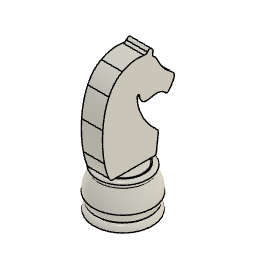
Knight (Autodesk Fusion 360 design; units mm, degrees)
Autodesk Fusion 360 part; units mm, degrees
sketch "Knight" plane through (0, 0, 0) normal (1, 0, 0) x (0, 1, 0)
  spline S0 degree 3 poles (14.2382, 40.3861) (12.0362, 41.9597) (10.374, 43.9521) (9.2277, 46.3988) knots 0 0 0 0 1 1 1 1
  spline S1 degree 3 poles (9.2277, 46.3988) (8.9049, 47.0874) (8.5729, 47.8295) (7.965, 48.2978) knots 0 0 0 0 1 1 1 1
  spline S2 degree 3 poles (7.965, 48.2978) (7.322, 48.7926) (6.9635, 49.21) (7.2909, 50.0977) knots 0 0 0 0 1 1 1 1
  spline S3 degree 3 poles (7.2909, 50.0977) (7.5575, 50.8193) (7.0766, 51.5377) (6.5098, 51.8929) knots 0 0 0 0 1 1 1 1
  spline S4 degree 3 poles (6.5098, 51.8929) (6.0189, 52.2004) (5.6055, 51.6131) (5.2649, 51.2248) knots 0 0 0 0 1 1 1 1
  spline S5 degree 3 poles (5.2649, 51.2248) (4.9137, 50.8259) (4.5287, 50.7565) (3.9698, 50.8517) knots 0 0 0 0 1 1 1 1
  spline S6 degree 3 poles (3.9698, 50.8517) (1.1063, 51.3405) (-1.6216, 50.8722) (-4.19, 49.5063) knots 0 0 0 0 1 1 1 1
  spline S7 degree 3 poles (-4.19, 49.5063) (-6.5984, 48.2257) (-8.1905, 46.2387) (-9.3084, 43.7854) knots 0 0 0 0 1 1 1 1
  spline S8 degree 3 poles (-9.3084, 43.7854) (-10.7411, 40.6434) (-11.4078, 37.3236) (-11.6307, 33.9177) knots 0 0 0 0 1 1 1 1
  spline S9 degree 3 poles (-11.6307, 33.9177) (-11.8748, 30.1792) (-11.7194, 26.4399) (-10.9898, 22.7563) knots 0 0 0 0 1 1 1 1
  spline S10 degree 3 poles (-10.9898, 22.7563) (-10.5982, 20.7798) (-10.1094, 18.8252) (-9.2118, 16.9824) knots 0 0 0 0 1 1 1 1
  spline S11 degree 3 poles (-9.2118, 16.9824) (-8.9036, 16.3467) (-8.5345, 16.0279) (-7.9848, 15.9194) knots 0 0 0 0 1 1 1 1
  line L0 (-7.9848, 15.9194) -> (7.9848, 15.9194)
  spline S12 degree 3 poles (7.9848, 15.9194) (8.4134, 16.0087) (8.5894, 16.2912) (8.6456, 16.8151) knots 0 0 0 0 1 1 1 1
  spline S13 degree 3 poles (8.6456, 16.8151) (8.8645, 18.8087) (9.1013, 20.7997) (9.3599, 22.7874) knots 0 0 0 0 1 1 1 1
  spline S14 degree 3 poles (9.3599, 22.7874) (9.4354, 23.3642) (9.264, 23.7505) (8.8347, 24.1526) knots 0 0 0 0 1 1 1 1
  spline S15 degree 3 poles (8.8347, 24.1526) (6.8755, 25.9809) (5.0611, 27.9362) (3.7779, 30.3254) knots 0 0 0 0 1 1 1 1
  spline S16 degree 3 poles (3.7779, 30.3254) (2.4874, 32.7311) (1.4793, 35.2208) (1.3887, 37.9983) knots 0 0 0 0 1 1 1 1
  spline S17 degree 3 poles (1.3887, 37.9983) (1.3742, 38.4243) (1.4688, 38.9918) (1.8332, 39.0242) knots 0 0 0 0 1 1 1 1
  spline S18 degree 3 poles (1.8332, 39.0242) (2.3214, 39.0678) (2.2076, 38.4659) (2.2751, 38.1147) knots 0 0 0 0 1 1 1 1
  spline S19 degree 3 poles (2.2751, 38.1147) (2.7103, 35.832) (3.9916, 35.1031) (6.2868, 35.656) knots 0 0 0 0 1 1 1 1
  spline S20 degree 3 poles (6.2868, 35.656) (8.2791, 36.1356) (10.2853, 36.4577) (11.9641, 34.6791) knots 0 0 0 0 1 1 1 1
  spline S21 degree 3 poles (11.9641, 34.6791) (12.1851, 34.4449) (12.914, 33.802) (13.5, 34.7611) knots 0 0 0 0 1 1 1 1
  spline S22 degree 3 poles (13.5, 34.7611) (13.9842, 35.5509) (14.6093, 36.2633) (15.0068, 37.1232) knots 0 0 0 0 1 1 1 1
  spline S23 degree 3 poles (15.0068, 37.1232) (15.6855, 38.5903) (15.5314, 39.4614) (14.2382, 40.3861) knots 0 0 0 0 1 1 1 1
  line L1 (-9.0666, 13.7263) -> (9.0666, 13.7263)
  spline S24 degree 3 poles (9.0666, 13.7263) (9.5051, 14.0021) (9.8597, 14.3719) (9.6268, 15.0432) knots 0 0 0 0 1 1 1 1
  spline S25 degree 3 poles (9.6268, 15.0432) (9.3398, 15.8694) (8.6274, 15.9131) (7.9084, 15.9117) knots 0 0 0 0 1 1 1 1
  spline S26 degree 3 poles (7.9084, 15.9117) (7.7682, 15.9117) (7.6299, 15.9064) (7.4897, 15.9078) knots 0 0 0 0 1 1 1 1
  spline S27 degree 3 poles (7.4897, 15.9078) (4.0157, 15.9117) (0.5404, 15.9223) (-2.9342, 15.9203) knots 0 0 0 0 1 1 1 1
  spline S28 degree 3 poles (-2.9342, 15.9203) (-4.7446, 15.9197) (-6.5551, 15.8932) (-8.3655, 15.8886) knots 0 0 0 0 1 1 1 1
  spline S29 degree 3 poles (-8.3655, 15.8886) (-9.1837, 15.8879) (-9.779, 15.5235) (-9.7836, 14.696) knots 0 0 0 0 1 1 1 1
  spline S30 degree 3 poles (-9.7836, 14.696) (-9.7863, 14.1403) (-9.4853, 13.8572) (-9.0666, 13.7263) knots 0 0 0 0 1 1 1 1
  line L2 (5.9758, 2.6224) -> (0, 2.6224)
  spline S31 degree 3 poles (10.1774, 0.0003) (10.5042, 0.001) (10.8839, -0.1015) (11.0042, 0.4012) knots 0 0 0 0 1 1 1 1
  spline S32 degree 3 poles (11.0042, 0.4012) (11.2509, 1.4258) (10.3401, 2.6177) (9.2877, 2.6158) knots 0 0 0 0 1 1 1 1
  line L3 (8.8867, 13.7263) -> (-8.8867, 13.7263)
  spline S33 degree 3 poles (-8.8867, 13.7263) (-9.3246, 13.5212) (-9.6474, 13.0919) (-9.9642, 12.5826) knots 0 0 0 0 1 1 1 1
  spline S34 degree 3 poles (-9.9642, 12.5826) (-10.3082, 12.0296) (-10.5734, 11.4515) (-10.8644, 10.8807) knots 0 0 0 0 1 1 1 1
  spline S35 degree 3 poles (-10.8644, 10.8807) (-12.108, 8.4578) (-11.977, 6.0381) (-10.8883, 3.5947) knots 0 0 0 0 1 1 1 1
  spline S36 degree 3 poles (-10.8883, 3.5947) (-10.6726, 3.1085) (-10.416, 2.7573) (-10.0363, 2.6224) knots 0 0 0 0 1 1 1 1
  line L4 (-10.0363, 2.6224) -> (-9.23, 2.6224)
  spline S37 degree 3 poles (-9.23, 2.6224) (-9.2267, 2.6224) (-9.2234, 2.6237) (-9.2221, 2.6244) knots 0 0 0 0 1 1 1 1
  spline S38 degree 3 poles (-9.2221, 2.6244) (-9.2214, 2.625) (-9.2214, 2.627) (-9.2214, 2.6283) knots 0 0 0 0 1 1 1 1
  spline S39 degree 3 poles (-9.2214, 2.6283) (-9.2181, 2.627) (-9.2161, 2.625) (-9.2141, 2.6244) knots 0 0 0 0 1 1 1 1
  spline S40 degree 3 poles (-9.2141, 2.6244) (-7.9018, 2.6244) (-6.5894, 2.6244) (-5.2771, 2.6244) knots 0 0 0 0 1 1 1 1
  spline S41 degree 2 poles (-5.2771, 2.6244) (-5.2771, 2.6237) (-5.2771, 2.6224) knots 0 0 0 1 1 1
  line L5 (-5.2771, 2.6224) -> (9.5118, 2.6224)
  spline S42 degree 3 poles (9.5118, 2.6224) (9.816, 2.7136) (10.037, 2.918) (10.2003, 3.2468) knots 0 0 0 0 1 1 1 1
  spline S43 degree 3 poles (10.2003, 3.2468) (10.6839, 4.2138) (11.0854, 5.1935) (11.1694, 6.31) knots 0 0 0 0 1 1 1 1
  spline S44 degree 3 poles (11.1694, 6.31) (11.3758, 9.0815) (10.3452, 11.431) (8.8867, 13.7263) knots 0 0 0 0 1 1 1 1
  line L6 (-9.2227, 2.6244) -> (-9.2227, 2.6224)
  line L7 (-9.2227, 2.6224) -> (-9.2115, 2.6224)
  line L8 (-9.2115, 2.6224) -> (-9.2154, 2.6244)
  line L9 (-9.2154, 2.6244) -> (-9.2221, 2.6244)
  line L10 (-9.2221, 2.6244) -> (-9.2227, 2.6244)
  line L11 (5.9758, 2.6224) -> (9.2877, 2.6158)
  spline S45 degree 3 poles (0, 0) (3.3925, -0.001) (6.785, -0.0011) (10.1774, 0.0003) knots 0.452185 0.452185 0.452185 0.452185 1 1 1 1
  spline S46 degree 3 poles (0, 0) (-3.3925, -0.001) (-6.785, -0.0011) (-10.1774, 0.0003) knots 0.452185 0.452185 0.452185 0.452185 1 1 1 1
  line L12 (-5.9758, 2.6224) -> (0, 2.6224)
  spline S47 degree 3 poles (-11.0042, 0.4012) (-11.2509, 1.4258) (-10.3401, 2.6177) (-9.2877, 2.6158) knots 0 0 0 0 1 1 1 1
  line L13 (-5.9758, 2.6224) -> (-9.2877, 2.6158)
  spline S48 degree 3 poles (-10.1774, 0.0003) (-10.5042, 0.001) (-10.8839, -0.1015) (-11.0042, 0.4012) knots 0 0 0 0 1 1 1 1
  line L14 (0, 0) -> (0, 50.9092)
  constraint coincident S45.start S46.start
  constraint coincident S6 L14.end
  constraint vertical L14
revolve "Revolve1" add sketch "Knight" angle 360 about axis through (0, 0, 0) along (0, 0, 1) contours L1 S24 S25 S26 S27 L3 L14 | L1 L2 L3 L5 S42 S43 S44 L14 | L2 S31 S32 L5 L11 S45 L14
extrude "Extrude1" add sketch "Knight" along normal mid plane 8 contours S0 S1 S2 S3 S4 S5 S6 L0 S12 S13 S14 S15 S16 S17 S18 S19 S20 S21 S22 S23 L14 | S6 S7 S8 S9 S10 S11 L0 S27 L14
named bodies: "knight"
